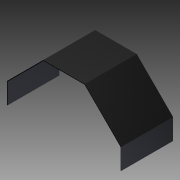
# Autodesk Inventor part: middle shell
Saved by Autodesk Inventor 2012 (Build 160160000, 160)
## iProperties
Created: 2011-11-30
Part Number: middle shell
Material: Default
Document SubType Name: Modeling
Designer: Antonella
Density: 1 g/cm^3
Author: Antonella
Autodesk Inventor part; units mm, degrees
ref_plane "YZ Plane" through (0, 0, 0) normal (1, 0, 0) x (0, 1, 0)
ref_plane "XZ Plane" through (0, 0, 0) normal (0, 1, 0) x (-1, 0, 0)
ref_plane "XY Plane" through (0, 0, 0) normal (0, 0, 1) x (1, 0, 0)
sketch "Sketch1" plane through (0, 0, 0) normal (0, 0, 1) x (1, 0, 0)
  line L0 (-391.16, 0) -> (391.16, 0) projected
  line L1 (0, -55.88) -> (0, 335.28) projected
  line L2 (-101.6, 279.4) -> (101.6, 279.4)
  line L3 (101.6, 279.4) -> (279.4, 101.6)
  line L4 (279.4, 101.6) -> (279.4, 0)
  line L5 (279.4, 0) -> (-279.4, 0) construction
  line L6 (-279.4, 0) -> (-279.4, 101.6)
  line L7 (-279.4, 101.6) -> (-101.6, 279.4)
  line L8 (-279.4, 101.6) -> (279.4, 101.6) construction
  line L9 (276.225, 100.2849) -> (100.2849, 276.225)
  line L10 (100.2849, 276.225) -> (-100.2849, 276.225)
  line L11 (-100.2849, 276.225) -> (-276.225, 100.2849)
  line L12 (-276.225, 100.2849) -> (-276.225, 0)
  line L13 (276.225, 0) -> (276.225, 100.2849)
  line L14 (-279.4, 0) -> (-276.225, 0)
  line L15 (276.225, 0) -> (279.4, 0)
  point P0 (0, 0)
  point P1 (-279.4, 50.8)
  point P2 (0, 0)
  point P3 (0, 279.4)
  dimension "d0" = 558.8
  dimension "d1" = 101.6
  dimension "d2" = 45
  dimension "d3" = 203.2
  dimension "d4" = 3.175
  dimension "d5" = 3.175
  dimension "d6" = 3.175
  dimension "d7" = 3.175
  constraints: 28 end point, 5 parallel, 3 collinear, 3 midpoint, 2 equal length, 2 perpendicular, 2 point on line, 1 coincident, 1 vertical alignment
  measures "d0" distance of L4.end L5.end
  measures "d1" distance of L3.end L4.end
  measures "d2" angle of L7 L8
  measures "d3" distance of L2.start L2.end
  measures "d4" distance between parallel lines of L4 L13
  measures "d5" distance between parallel lines of L2 L10
  measures "d6" distance between parallel lines of L3 L9
  measures "d7" distance between parallel lines of L7 L11
extrude "Extrusion1" add sketch "Sketch1" along normal mid plane 254 contours L6 L7 L2 L1 L10 L11 L12 L0 | L13 L9 L10 L1 L2 L3 L4 L0
equation "\"d5\" = d4"
equation "\"d6\" = d4"
equation "\"d7\" = d4"
body "Solid1"
